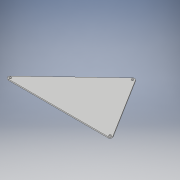
# Autodesk Inventor part: test
Saved by Autodesk Inventor 2019 (Build 230136000, 136)
## iProperties
Created: 2021-02-18
Part Number: test
Material: 一般
Document SubType Name: Modeling
Designer: wasd5
Density: 1 g/cm^3
Appearance: 預設
Author: wasd5
Autodesk Inventor part; units mm, degrees
ref_plane "YZ Plane" through (0, 0, 0) normal (1, 0, 0) x (0, 1, 0)
ref_plane "XZ Plane" through (0, 0, 0) normal (0, 1, 0) x (-1, 0, 0)
ref_plane "XY Plane" through (0, 0, 0) normal (0, 0, 1) x (1, 0, 0)
sketch "草圖2" plane through (0, 0, 0) normal (0, 1, 0) x (-1, 0, 0)
  line L0 (-295.9066, -280.8973) -> (0, 0) construction
  line L1 (0, 0) -> (-471, 0) construction
  arc A0 (-471, 10) -> (-479.4863, -5.2898) centre (-471, 0) ccw
  arc A1 (6.8847, -7.2526) -> (0, 10) centre (0, 0) ccw
  line L2 (-471, 10) -> (0, 10)
  line L3 (-479.4863, -5.2898) -> (-304.3929, -286.1871)
  line L4 (-471, 0) -> (-295.9066, -280.8973) construction
  arc A2 (-304.3929, -286.1871) -> (-289.0218, -288.1499) centre (-295.9066, -280.8973) ccw
  line L5 (6.8847, -7.2526) -> (-289.0218, -288.1499)
  circle A3 centre (-471, 0) radius 5
  circle A4 centre (0, 0) radius 5
  circle A5 centre (-295.9066, -280.8973) radius 5
  dimension "d11" = 20
  dimension "hole" = 10
  dimension "center_distance1" = 471
  dimension "center_distance3" = 331
  dimension "center_distance2" = 408
  constraints: 12 end point, 7 coincident, 6 centre point, 6 point on circle, 6 tangent, 4 equal radius, 1 horizontal
  measures "d11" diameter of A0
  measures "hole" diameter of A3
  measures "center_distance1" distance of L1.start L1.end
  measures "center_distance3" distance of L4.start L4.end
  measures "center_distance2" distance of L4.end L1.start
extrude "擠出2" add sketch "草圖2" along normal blind 5
equation "\"d11\" = 2 * hole"
